Autodesk Fusion 360 part; units mm, degrees
note: some values were not read from the file. Chosen so that the rebuilt part matches the saved one: which pieces of a blend or face edit are solid. Set by a fixed rule: which sketch regions a step uses.
(part 2 of 3)
  spline S367 degree 3 poles (41.2974, -19.9603) (42.5718, -19.3541) (43.9034, -18.9073) (45.3289, -18.8182) knots 0 0 0 0 1 1 1 1
  spline S368 degree 3 poles (45.3289, -18.8182) (46.5961, -18.7389) (47.768, -19.0007) (48.7702, -19.8267) knots 0 0 0 0 1 1 1 1
  spline S369 degree 3 poles (48.7702, -19.8267) (49.4912, -20.4209) (49.8984, -21.1818) (49.9641, -22.1189) knots 0 0 0 0 1 1 1 1
  spline S370 degree 3 poles (49.9641, -22.1189) (49.9692, -22.1925) (49.9778, -22.2661) (49.9884, -22.3391) knots 0 0 0 0 1 1 1 1
  spline S371 degree 3 poles (49.9884, -22.3391) (49.9927, -22.3689) (50.0063, -22.3974) (50.0157, -22.4264) knots 0 0 0 0 1 1 1 1
  spline S372 degree 3 poles (50.0157, -22.4264) (50.0388, -22.4327) (50.0618, -22.439) (50.0849, -22.4264) knots 0 0 0 0 1 1 1 1
  spline S373 degree 3 poles (103.7652, -25.3114) (103.6868, -24.832) (103.6099, -23.932) (103.3842, -23.071) knots 0 0 0 0 1 1 1 1
  spline S374 degree 3 poles (103.3842, -23.071) (102.9323, -21.3472) (101.8898, -20.1667) (100.0685, -19.7927) knots 0 0 0 0 1 1 1 1
  spline S375 degree 3 poles (100.0685, -19.7927) (97.9906, -19.366) (96.1141, -19.7496) (94.434, -21.0869) knots 0 0 0 0 1 1 1 1
  spline S376 degree 3 poles (94.434, -21.0869) (92.8843, -22.3203) (91.7133, -23.8561) (90.75, -25.561) knots 0 0 0 0 1 1 1 1
  spline S377 degree 3 poles (90.75, -25.561) (88.9387, -28.7669) (87.8127, -32.2136) (87.2249, -35.8387) knots 0 0 0 0 1 1 1 1
  spline S378 degree 3 poles (87.2249, -35.8387) (86.9707, -37.4063) (86.8196, -38.9843) (87.089, -40.569) knots 0 0 0 0 1 1 1 1
  spline S379 degree 3 poles (87.089, -40.569) (87.4308, -42.5797) (88.511, -43.9928) (90.5089, -44.5579) knots 0 0 0 0 1 1 1 1
  spline S380 degree 3 poles (90.5089, -44.5579) (92.2381, -45.047) (93.88, -44.7412) (95.3927, -43.7705) knots 0 0 0 0 1 1 1 1
  spline S381 degree 3 poles (95.3927, -43.7705) (96.8708, -42.822) (98.0012, -41.534) (98.9616, -40.0853) knots 0 0 0 0 1 1 1 1
  spline S382 degree 3 poles (98.9616, -40.0853) (100.7237, -37.4275) (101.8987, -34.5089) (102.7607, -31.4561) knots 0 0 0 0 1 1 1 1
  spline S383 degree 3 poles (102.7607, -31.4561) (103.2897, -29.5826) (103.6858, -27.6833) (103.7652, -25.3114) knots 0 0 0 0 1 1 1 1
  spline S384 degree 3 poles (46.0065, -19.6332) (44.9669, -19.627) (44.0162, -19.8508) (43.1126, -20.2652) knots 0 0 0 0 1 1 1 1
  spline S385 degree 3 poles (43.1126, -20.2652) (41.2513, -21.1186) (39.7466, -22.4329) (38.4102, -23.9545) knots 0 0 0 0 1 1 1 1
  spline S386 degree 3 poles (38.4102, -23.9545) (36.618, -25.9951) (35.2451, -28.3068) (34.0956, -30.753) knots 0 0 0 0 1 1 1 1
  spline S387 degree 3 poles (34.0956, -30.753) (32.774, -33.5658) (31.7466, -36.4734) (31.4534, -39.5941) knots 0 0 0 0 1 1 1 1
  spline S388 degree 3 poles (31.4534, -39.5941) (31.3429, -40.7711) (31.3958, -41.9355) (31.8603, -43.0504) knots 0 0 0 0 1 1 1 1
  spline S389 degree 3 poles (31.8603, -43.0504) (32.3368, -44.1941) (33.2068, -44.7345) (34.4271, -44.7672) knots 0 0 0 0 1 1 1 1
  spline S390 degree 3 poles (34.4271, -44.7672) (35.6477, -44.7998) (36.7623, -44.4442) (37.8098, -43.852) knots 0 0 0 0 1 1 1 1
  spline S391 degree 3 poles (37.8098, -43.852) (40.0373, -42.5928) (41.8175, -40.8319) (43.3761, -38.8332) knots 0 0 0 0 1 1 1 1
  spline S392 degree 3 poles (43.3761, -38.8332) (44.1228, -37.8756) (44.8434, -36.8973) (45.2618, -35.7354) knots 0 0 0 0 1 1 1 1
  spline S393 degree 3 poles (45.2618, -35.7354) (46.3267, -32.778) (47.4017, -29.8244) (48.4649, -26.8664) knots 0 0 0 0 1 1 1 1
  spline S394 degree 3 poles (48.4649, -26.8664) (48.8497, -25.7959) (49.3037, -24.7413) (49.4107, -23.5928) knots 0 0 0 0 1 1 1 1
  spline S395 degree 3 poles (49.4107, -23.5928) (49.6232, -21.3105) (48.1691, -19.514) (46.0065, -19.6332) knots 0 0 0 0 1 1 1 1
  spline S396 degree 3 poles (84.1667, -10.1913) (84.1729, -8.6259) (85.3768, -7.4326) (86.9503, -7.4324) knots 0 0 0 0 1 1 1 1
  spline S397 degree 3 poles (86.9503, -7.4324) (88.5314, -7.4321) (89.7239, -8.6369) (89.7211, -10.2316) knots 0 0 0 0 1 1 1 1
  spline S398 degree 3 poles (89.7211, -10.2316) (89.7183, -11.8206) (88.5136, -13.0149) (86.9258, -13.0029) knots 0 0 0 0 1 1 1 1
  spline S399 degree 3 poles (86.9258, -13.0029) (85.3374, -12.9908) (84.1605, -11.7915) (84.1667, -10.1913) knots 0 0 0 0 1 1 1 1
  spline S400 degree 3 poles (128.8614, -26.1716) (128.8153, -28.284) (128.276, -30.6235) (127.5153, -32.9166) knots 0 0 0 0 1 1 1 1
  spline S401 degree 3 poles (127.5153, -32.9166) (126.5931, -35.6965) (125.3817, -38.3368) (123.61, -40.6911) knots 0 0 0 0 1 1 1 1
  spline S402 degree 3 poles (123.61, -40.6911) (122.5647, -42.0801) (121.3489, -43.2903) (119.806, -44.129) knots 0 0 0 0 1 1 1 1
  spline S403 degree 3 poles (119.806, -44.129) (118.0331, -45.0928) (115.4801, -45.0947) (113.845, -43.5861) knots 0 0 0 0 1 1 1 1
  spline S404 degree 3 poles (113.845, -43.5861) (112.9324, -42.7442) (112.3341, -41.7221) (111.9863, -40.5443) knots 0 0 0 0 1 1 1 1
  spline S405 degree 3 poles (111.9863, -40.5443) (111.834, -40.0287) (111.687, -39.5095) (111.5818, -38.983) knots 0 0 0 0 1 1 1 1
  spline S406 degree 3 poles (111.5818, -38.983) (111.5353, -38.7499) (111.5424, -38.4751) (111.6206, -38.2527) knots 0 0 0 0 1 1 1 1
  spline S407 degree 3 poles (111.6206, -38.2527) (113.0797, -34.1034) (114.5515, -29.9585) (116.0281, -25.8153) knots 0 0 0 0 1 1 1 1
  spline S408 degree 3 poles (116.0281, -25.8153) (116.1079, -25.5914) (116.2291, -25.3728) (116.3717, -25.182) knots 0 0 0 0 1 1 1 1
  spline S409 degree 3 poles (116.3717, -25.182) (117.2705, -23.9794) (118.185, -22.7878) (119.3159, -21.7871) knots 0 0 0 0 1 1 1 1
  spline S410 degree 3 poles (119.3159, -21.7871) (120.4047, -20.8235) (121.5941, -20.0336) (123.056, -19.7578) knots 0 0 0 0 1 1 1 1
  spline S411 degree 3 poles (123.056, -19.7578) (123.9276, -19.5934) (124.8028, -19.5937) (125.6676, -19.8061) knots 0 0 0 0 1 1 1 1
  spline S412 degree 3 poles (125.6676, -19.8061) (126.9085, -20.111) (127.6838, -20.9266) (128.1613, -22.0809) knots 0 0 0 0 1 1 1 1
  spline S413 degree 3 poles (128.1613, -22.0809) (128.6621, -23.2915) (128.8638, -24.5521) (128.8614, -26.1716) knots 0 0 0 0 1 1 1 1
  spline S414 degree 3 poles (138.7712, -30.0038) (139.2283, -29.0291) (139.6235, -28.0968) (140.0927, -27.2034) knots 0 0 0 0 1 1 1 1
  spline S415 degree 3 poles (140.0927, -27.2034) (141.2378, -25.0227) (142.6739, -23.0631) (144.619, -21.5155) knots 0 0 0 0 1 1 1 1
  spline S416 degree 3 poles (144.619, -21.5155) (145.6449, -20.6992) (146.7387, -19.9808) (148.0608, -19.7806) knots 0 0 0 0 1 1 1 1
  spline S417 degree 3 poles (148.0608, -19.7806) (148.7512, -19.6761) (149.4761, -19.6581) (150.1687, -19.7408) knots 0 0 0 0 1 1 1 1
  spline S418 degree 3 poles (150.1687, -19.7408) (151.3327, -19.8797) (152.1161, -20.7367) (152.2726, -21.9102) knots 0 0 0 0 1 1 1 1
  spline S419 degree 3 poles (152.2726, -21.9102) (152.4727, -23.4101) (151.9809, -24.7224) (151.122, -25.9174) knots 0 0 0 0 1 1 1 1
  spline S420 degree 3 poles (151.122, -25.9174) (149.935, -27.569) (148.2949, -28.6145) (146.4395, -29.3662) knots 0 0 0 0 1 1 1 1
  spline S421 degree 3 poles (146.4395, -29.3662) (144.4026, -30.1915) (142.2832, -30.356) (140.1191, -30.1628) knots 0 0 0 0 1 1 1 1
  spline S422 degree 3 poles (140.1191, -30.1628) (139.7002, -30.1254) (139.2833, -30.0649) (138.7712, -30.0038) knots 0 0 0 0 1 1 1 1
  spline S423 degree 3 poles (103.7652, -25.3302) (103.6859, -27.7021) (103.2897, -29.6014) (102.7607, -31.4749) knots 0 0 0 0 1 1 1 1
  spline S424 degree 3 poles (102.7607, -31.4749) (101.8987, -34.5277) (100.7238, -37.4463) (98.9617, -40.1041) knots 0 0 0 0 1 1 1 1
  spline S425 degree 3 poles (98.9617, -40.1041) (98.0012, -41.5528) (96.8709, -42.8408) (95.3927, -43.7893) knots 0 0 0 0 1 1 1 1
  spline S426 degree 3 poles (95.3927, -43.7893) (93.8801, -44.76) (92.2382, -45.0658) (90.509, -44.5767) knots 0 0 0 0 1 1 1 1
  spline S427 degree 3 poles (90.509, -44.5767) (88.511, -44.0116) (87.4309, -42.5985) (87.089, -40.5878) knots 0 0 0 0 1 1 1 1
  spline S428 degree 3 poles (87.089, -40.5878) (86.8196, -39.0031) (86.9707, -37.4251) (87.2249, -35.8575) knots 0 0 0 0 1 1 1 1
  spline S429 degree 3 poles (87.2249, -35.8575) (87.8128, -32.2324) (88.9387, -28.7857) (90.7501, -25.5798) knots 0 0 0 0 1 1 1 1
  spline S430 degree 3 poles (90.7501, -25.5798) (91.7133, -23.8749) (92.8844, -22.3391) (94.4341, -21.1057) knots 0 0 0 0 1 1 1 1
  spline S431 degree 3 poles (94.4341, -21.1057) (96.1142, -19.7684) (97.9907, -19.3848) (100.0686, -19.8115) knots 0 0 0 0 1 1 1 1
  spline S432 degree 3 poles (100.0686, -19.8115) (101.8899, -20.1855) (102.9323, -21.366) (103.3842, -23.0898) knots 0 0 0 0 1 1 1 1
  spline S433 degree 3 poles (103.3842, -23.0898) (103.61, -23.9508) (103.6869, -24.8508) (103.7652, -25.3302) knots 0 0 0 0 1 1 1 1
  spline S434 degree 3 poles (46.0066, -19.652) (48.1692, -19.5328) (49.6232, -21.3293) (49.4107, -23.6116) knots 0 0 0 0 1 1 1 1
  spline S435 degree 3 poles (49.4107, -23.6116) (49.3038, -24.7601) (48.8497, -25.8147) (48.4649, -26.8852) knots 0 0 0 0 1 1 1 1
  spline S436 degree 3 poles (48.4649, -26.8852) (47.4017, -29.8432) (46.3267, -32.7968) (45.2618, -35.7542) knots 0 0 0 0 1 1 1 1
  spline S437 degree 3 poles (45.2618, -35.7542) (44.8434, -36.9161) (44.1228, -37.8944) (43.3761, -38.852) knots 0 0 0 0 1 1 1 1
  spline S438 degree 3 poles (43.3761, -38.852) (41.8175, -40.8507) (40.0373, -42.6116) (37.8099, -43.8708) knots 0 0 0 0 1 1 1 1
  spline S439 degree 3 poles (37.8099, -43.8708) (36.7624, -44.463) (35.6477, -44.8186) (34.4271, -44.786) knots 0 0 0 0 1 1 1 1
  spline S440 degree 3 poles (34.4271, -44.786) (33.2068, -44.7533) (32.3368, -44.213) (31.8603, -43.0692) knots 0 0 0 0 1 1 1 1
  spline S441 degree 3 poles (31.8603, -43.0692) (31.3958, -41.9543) (31.3429, -40.7899) (31.4535, -39.6129) knots 0 0 0 0 1 1 1 1
  spline S442 degree 3 poles (31.4535, -39.6129) (31.7466, -36.4922) (32.774, -33.5846) (34.0957, -30.7718) knots 0 0 0 0 1 1 1 1
  spline S443 degree 3 poles (34.0957, -30.7718) (35.2451, -28.3256) (36.618, -26.0139) (38.4102, -23.9733) knots 0 0 0 0 1 1 1 1
  spline S444 degree 3 poles (38.4102, -23.9733) (39.7466, -22.4517) (41.2513, -21.1374) (43.1126, -20.284) knots 0 0 0 0 1 1 1 1
  spline S445 degree 3 poles (43.1126, -20.284) (44.0162, -19.8697) (44.967, -19.6458) (46.0066, -19.652) knots 0 0 0 0 1 1 1 1
extrude "Extrude3" add sketch "Sketch3" along normal blind 6.35 contours S23 S24 S25 S26 S27 S28 S29 S30 S31 S32 S33 S34 S35 S36 S37 S38 S39 S40 S41 S42 S43 S44 S45 S214 S215 S216 S217 S218 S219 S220 S221 S222 S223 S224 S225 S226 S227 S228 S229 S230 S231 S232 S233 S234 S235 L21 | S0 L2 S1 S2 S3 S4 S5 S6 S7 S8 S9 S10 L3 S11 L4 S12 S13 S14 S15 L5 S16 S17 S18 S19 S20 S21 S178 S179 S180 S181 S182 S183 L16 S184 S185 S186 S187 L17 S188 L18 S189 S190 S191 S192 S193 S194 S195 S196 S197 S198 L19 S199 L20 | S46 S47 S48 S49 S50 S51 S52 S53 S54 S55 S56 S57 S58 S59 S60 S61 S62 S63 S64 S65 S66 S67 S68 S69 S70 S71 S72 S73 S74 S75 S76 S77 S78 S79 S80 S81 S82 S83 S84 S85 S86 S87 S88 S89 S90 S91 S92 S93 S94 S95 S96 S97 S98 S99 S100 S101 S102 S103 S104 S105 S106 S107 S108 S109 S111 S112 S113 S114 S115 S116 S117 S118 S119 S120 S121 S122 S123 S124 S125 S126 S127 S128 L9 S129 S130 S131 S132 L10 S133 S134 S135 S136 S137 S138 S139 S140 S141 S142 L11 S143 S144 S145 L12 S146 S147 S148 S149 S150 S151 S152 S153 S154 S155 L13 S156 L14 S157 S158 S159 S160 S161 S162 S163 S164 S165 S166 S167 S168 S169 S170 S171 S172 S173 S245 S246 S247 S248 S249 S250 S251 S252 S253 S254 S255 S256 S257 S258 S259 S260 S261 L22 S262 L23 S263 S264 S265 S266 S267 S268 S269 S270 S271 S272 L24 S273 S274 S275 L25 S276 S277 S278 S279 S280 S281 S282 S283 S284 S285 L26 S286 S287 S288 S289 L27 S290 S291 S292 S293 S294 S295 S296 S297 S298 S299 S300 S301 S302 S303 S304 S305 S306 S307 S309 S310 S311 S312 S313 S314 S315 S316 S317 S318 S319 S320 S321 S322 S323 S324 S325 S326 S327 S328 S329 S330 S331 S332 S333 S334 S335 S336 S337 S338 S339 S340 S341 S342 S343 S344 S345 S346 S347 S348 S349 S350 S351 S352 S353 S354 S355 S356 S357 S358 S359 S360 S361 S362 S363 S364 S365 S366 S367 S368 S369 S370 S371 | S174 S175 S176 S177 S396 S397 S398 S399 makes body 1 at (108.0941, -40.2976, 0) makes body 2 at (65.2632, -12.3093, 0) makes body 3 at (138.449, -28.0132, 0) makes body 4 at (84.2074, -10.7088, 2.8222)
sketch "Sketch4" plane through (0, 0, 0) normal (0, 0, 1) x (1, 0, 0)
  line L0 (0, 0) -> (156.0835, 0)
  line L1 (156.0835, 0) -> (156.0835, -61.3211)
  line L2 (156.0835, -61.3211) -> (0, -61.3211)
  line L3 (0, -61.3211) -> (0, 0)
  constraint horizontal L0
  constraint vertical L1
  constraint horizontal L2
  constraint vertical L3
  constraint coincident L0.start L3.end
extrude "Extrude4" add sketch "Sketch4" against normal blind 6.35 bodies 1 2 3 4
fillet "Fillet1" radius 6.35 4 edges at (0, -61.3211, -3.175) (156.0835, -61.3211, -3.175) (156.0835, 0, -3.175) (0, 0, -3.175) on bodies 1
sketch "Sketch1" plane through (0, 0, 0) normal (0, 0, 1) x (1, 0, 0)
  line L0 (156.0195, -23.5976) -> (156.0195, -61.341)
  line L1 (156.0195, -61.341) -> (108.4773, -61.341)
  spline S0 degree 3 poles (108.4773, -61.341) (108.5491, -61.0596) (108.6209, -60.7783) (108.7043, -60.4516) knots 0 0 0 0 1 1 1 1
  line L2 (108.7043, -60.4516) -> (103.7692, -60.4516)
  spline S1 degree 3 poles (103.7692, -60.4516) (106.1753, -53.6131) (108.5658, -46.8189) (110.9796, -39.9584) knots 0 0 0 0 1 1 1 1
  spline S2 degree 3 poles (110.9796, -39.9584) (111.1778, -40.6135) (111.3001, -41.1945) (111.5257, -41.7321) knots 0 0 0 0 1 1 1 1
  spline S3 degree 3 poles (111.5257, -41.7321) (112.4488, -43.9326) (114.0522, -45.3171) (116.4762, -45.532) knots 0 0 0 0 1 1 1 1
  spline S4 degree 3 poles (116.4762, -45.532) (118.5105, -45.7123) (120.4877, -45.3426) (122.343, -44.485) knots 0 0 0 0 1 1 1 1
  spline S5 degree 3 poles (122.343, -44.485) (125.9058, -42.8382) (128.6456, -40.264) (130.6312, -36.8985) knots 0 0 0 0 1 1 1 1
  spline S6 degree 3 poles (130.6312, -36.8985) (132.3382, -34.0054) (133.3231, -30.9198) (132.9158, -27.5036) knots 0 0 0 0 1 1 1 1
  spline S7 degree 3 poles (132.9158, -27.5036) (132.7164, -25.831) (132.2982, -24.2283) (131.4403, -22.7614) knots 0 0 0 0 1 1 1 1
  spline S8 degree 3 poles (131.4403, -22.7614) (129.2488, -19.0142) (125.0975, -18.1221) (121.9017, -19.2309) knots 0 0 0 0 1 1 1 1
  spline S9 degree 3 poles (121.9017, -19.2309) (119.7817, -19.9664) (118.1223, -21.3511) (116.8137, -23.1628) knots 0 0 0 0 1 1 1 1
  spline S10 degree 3 poles (116.8137, -23.1628) (116.7552, -23.2438) (116.6934, -23.3224) (116.6331, -23.4021) knots 0 0 0 0 1 1 1 1
  line L3 (116.6331, -23.4021) -> (116.5718, -23.3725)
  spline S11 degree 3 poles (116.5718, -23.3725) (116.9751, -22.1176) (117.3783, -20.8626) (117.794, -19.5691) knots 0 0 0 0 1 1 1 1
  line L4 (117.794, -19.5691) -> (117.39, -19.5691)
  spline S12 degree 3 poles (117.39, -19.5691) (116.1524, -19.5691) (114.9147, -19.5691) (113.677, -19.5691) knots 0 0 0 0 1 1 1 1
  spline S13 degree 3 poles (113.677, -19.5691) (112.0374, -19.5691) (110.3977, -19.567) (108.7581, -19.5739) knots 0 0 0 0 1 1 1 1
  spline S14 degree 3 poles (108.7581, -19.5739) (108.6477, -19.5743) (108.4711, -19.6131) (108.4397, -19.6844) knots 0 0 0 0 1 1 1 1
  spline S15 degree 3 poles (108.4397, -19.6844) (108.3413, -19.9076) (108.2979, -20.1549) (108.2252, -20.4221) knots 0 0 0 0 1 1 1 1
  line L5 (108.2252, -20.4221) -> (113.6878, -20.4221)
  spline S16 degree 3 poles (113.6878, -20.4221) (113.6473, -20.5473) (113.6177, -20.6465) (113.5834, -20.7441) knots 0 0 0 0 1 1 1 1
  spline S17 degree 3 poles (113.5834, -20.7441) (108.9605, -33.8922) (104.3365, -47.04) (99.7194, -60.1902) knots 0 0 0 0 1 1 1 1
  spline S18 degree 3 poles (99.7194, -60.1902) (99.6414, -60.4125) (99.533, -60.4699) (99.3115, -60.4681) knots 0 0 0 0 1 1 1 1
  spline S19 degree 3 poles (99.3115, -60.4681) (98.0845, -60.4581) (96.8573, -60.46) (95.6303, -60.4696) knots 0 0 0 0 1 1 1 1
  spline S20 degree 3 poles (95.6303, -60.4696) (95.5302, -60.4704) (95.3717, -60.5363) (95.342, -60.6118) knots 0 0 0 0 1 1 1 1
  spline S21 degree 3 poles (95.342, -60.6118) (95.2508, -60.8445) (95.2089, -61.0965) (95.1478, -61.341) knots 0 0 0 0 1 1 1 1
  line L6 (95.1478, -61.341) -> (0, -61.341)
  line L7 (0, -61.341) -> (0, 0)
  spline S22 degree 3 poles (0, 0) (52.0065, 0) (104.013, 0) (156.0195, 0) knots 0 0 0 0 1 1 1 1
  line L8 (156.0195, 0) -> (156.0195, -22.8998)
  spline S23 degree 3 poles (156.0195, -22.8998) (156.0019, -22.8646) (155.9715, -22.8305) (155.9685, -22.7942) knots 0 0 0 0 1 1 1 1
  spline S24 degree 3 poles (155.9685, -22.7942) (155.8892, -21.8192) (155.4189, -21.052) (154.6851, -20.4397) knots 0 0 0 0 1 1 1 1
  spline S25 degree 3 poles (154.6851, -20.4397) (153.4053, -19.3719) (151.8701, -18.9809) (150.2562, -18.8437) knots 0 0 0 0 1 1 1 1
  spline S26 degree 3 poles (150.2562, -18.8437) (147.8053, -18.6354) (145.5366, -19.2454) (143.4312, -20.4739) knots 0 0 0 0 1 1 1 1
  spline S27 degree 3 poles (143.4312, -20.4739) (139.1005, -23.0008) (136.0205, -26.6341) (134.0532, -31.2182) knots 0 0 0 0 1 1 1 1
  spline S28 degree 3 poles (134.0532, -31.2182) (133.1018, -33.4352) (132.6126, -35.7441) (132.9818, -38.1701) knots 0 0 0 0 1 1 1 1
  spline S29 degree 3 poles (135.3221, -43.0231) (136.8021, -44.5156) (138.6131, -45.3113) (140.7013, -45.5057) knots 0 0 0 0 1 1 1 1
  spline S30 degree 3 poles (140.7013, -45.5057) (143.1519, -45.7339) (145.4639, -45.3818) (147.6206, -44.0951) knots 0 0 0 0 1 1 1 1
  spline S31 degree 3 poles (147.6206, -44.0951) (149.696, -42.8569) (151.1962, -41.1095) (152.41, -39.0493) knots 0 0 0 0 1 1 1 1
  spline S32 degree 3 poles (152.41, -39.0493) (152.1937, -38.9254) (151.9691, -38.7968) (151.7296, -38.6596) knots 0 0 0 0 1 1 1 1
  spline S33 degree 3 poles (151.7296, -38.6596) (151.52, -38.9343) (151.3182, -39.1785) (151.1384, -39.4379) knots 0 0 0 0 1 1 1 1
  spline S34 degree 3 poles (151.1384, -39.4379) (150.286, -40.6676) (149.3449, -41.8167) (148.1741, -42.7628) knots 0 0 0 0 1 1 1 1
  spline S35 degree 3 poles (148.1741, -42.7628) (146.3193, -44.2615) (144.246, -45.0682) (141.8277, -44.718) knots 0 0 0 0 1 1 1 1
  spline S36 degree 3 poles (141.8277, -44.718) (139.955, -44.4468) (138.4938, -43.5447) (137.642, -41.8068) knots 0 0 0 0 1 1 1 1
  spline S37 degree 3 poles (137.642, -41.8068) (137.1687, -40.8411) (137.0345, -39.7935) (137.0087, -38.7285) knots 0 0 0 0 1 1 1 1
  spline S38 degree 3 poles (137.0087, -38.7285) (136.9596, -36.7106) (137.328, -34.757) (137.9094, -32.836) knots 0 0 0 0 1 1 1 1
  spline S39 degree 3 poles (137.9094, -32.836) (138.1099, -32.1735) (138.3185, -31.5134) (138.503, -30.9178) knots 0 0 0 0 1 1 1 1
  spline S40 degree 3 poles (138.503, -30.9178) (139.7894, -30.9729) (141.0146, -31.0989) (142.2347, -31.0619) knots 0 0 0 0 1 1 1 1
  spline S41 degree 3 poles (142.2347, -31.0619) (144.493, -30.9934) (146.7045, -30.5779) (148.8648, -29.9105) knots 0 0 0 0 1 1 1 1
  spline S42 degree 3 poles (148.8648, -29.9105) (150.5076, -29.403) (152.0871, -28.7496) (153.4759, -27.7167) knots 0 0 0 0 1 1 1 1
  spline S43 degree 3 poles (153.4759, -27.7167) (154.6089, -26.874) (155.5238, -25.8533) (155.8582, -24.4251) knots 0 0 0 0 1 1 1 1
  spline S44 degree 3 poles (155.8582, -24.4251) (155.9223, -24.1517) (155.9663, -23.8735) (156.0195, -23.5976) knots 0 0 0 0 1 1 1 1
  spline S45 degree 3 poles (50.0849, -22.4452) (50.0619, -22.439) (50.0388, -22.4327) (50.0158, -22.4265) knots 0 0 0 0 1 1 1 1
  spline S46 degree 3 poles (50.0158, -22.4265) (50.0064, -22.3974) (49.9927, -22.3689) (49.9884, -22.3392) knots 0 0 0 0 1 1 1 1
  spline S47 degree 3 poles (49.9884, -22.3392) (49.9779, -22.2661) (49.9693, -22.1925) (49.9641, -22.1189) knots 0 0 0 0 1 1 1 1
  spline S48 degree 3 poles (49.9641, -22.1189) (49.8984, -21.1818) (49.4912, -20.4209) (48.7702, -19.8267) knots 0 0 0 0 1 1 1 1
  spline S49 degree 3 poles (48.7702, -19.8267) (47.7681, -19.0007) (46.5961, -18.7389) (45.3289, -18.8182) knots 0 0 0 0 1 1 1 1
  spline S50 degree 3 poles (45.3289, -18.8182) (43.9034, -18.9073) (42.5718, -19.3541) (41.2975, -19.9603) knots 0 0 0 0 1 1 1 1
  spline S51 degree 3 poles (41.2975, -19.9603) (37.4617, -21.785) (34.2471, -24.4068) (31.5841, -27.6967) knots 0 0 0 0 1 1 1 1
  spline S52 degree 3 poles (31.5841, -27.6967) (29.8681, -29.8167) (28.5608, -32.172) (27.7761, -34.8009) knots 0 0 0 0 1 1 1 1
  spline S53 degree 3 poles (27.7761, -34.8009) (27.6548, -35.2071) (27.6013, -35.6146) (27.2979, -35.9909) knots 0 0 0 0 1 1 1 1
  spline S54 degree 3 poles (27.2979, -35.9909) (26.7981, -36.6105) (26.4452, -37.3469) (26.0145, -38.024) knots 0 0 0 0 1 1 1 1
  spline S55 degree 3 poles (26.0145, -38.024) (24.3785, -40.5957) (22.1935, -42.5594) (19.4153, -43.8207) knots 0 0 0 0 1 1 1 1
  spline S56 degree 3 poles (19.4153, -43.8207) (16.336, -45.2186) (13.1649, -45.1705) (10.0109, -44.1478) knots 0 0 0 0 1 1 1 1
  spline S57 degree 3 poles (10.0109, -44.1478) (7.3021, -43.2695) (5.6053, -41.3794) (4.9304, -38.5933) knots 0 0 0 0 1 1 1 1
  spline S58 degree 3 poles (4.9304, -38.5933) (4.4781, -36.726) (4.5193, -34.842) (4.7229, -32.9543) knots 0 0 0 0 1 1 1 1
  spline S59 degree 3 poles (4.7229, -32.9543) (5.0136, -30.2599) (5.5761, -27.6183) (6.3535, -25.0241) knots 0 0 0 0 1 1 1 1
  spline S60 degree 3 poles (6.3535, -25.0241) (7.7161, -20.4766) (9.4965, -16.1067) (12.0128, -12.064) knots 0 0 0 0 1 1 1 1
  spline S61 degree 3 poles (12.0128, -12.064) (13.6498, -9.4342) (15.5983, -7.0752) (18.1065, -5.2075) knots 0 0 0 0 1 1 1 1
  spline S62 degree 3 poles (18.1065, -5.2075) (21.6115, -2.5974) (25.4024, -2.3618) (29.3636, -3.8873) knots 0 0 0 0 1 1 1 1
  spline S63 degree 3 poles (29.3636, -3.8873) (31.4072, -4.6744) (32.7504, -6.1919) (33.298, -8.3429) knots 0 0 0 0 1 1 1 1
  spline S64 degree 3 poles (33.298, -8.3429) (33.6344, -9.6642) (33.5355, -11.0084) (33.4161, -12.3468) knots 0 0 0 0 1 1 1 1
  spline S65 degree 3 poles (33.4161, -12.3468) (33.3593, -12.9843) (33.2661, -13.6185) (33.1895, -14.2539) knots 0 0 0 0 1 1 1 1
  spline S66 degree 3 poles (33.1895, -14.2539) (33.924, -14.3486) (33.9218, -14.3478) (34.1497, -13.71) knots 0 0 0 0 1 1 1 1
  spline S67 degree 3 poles (34.1497, -13.71) (35.1509, -10.908) (36.1535, -8.1065) (37.1555, -5.3048) knots 0 0 0 0 1 1 1 1
  spline S68 degree 3 poles (37.1555, -5.3048) (37.4387, -4.513) (37.7215, -3.721) (38.014, -2.9026) knots 0 0 0 0 1 1 1 1
  spline S69 degree 3 poles (38.014, -2.9026) (37.8301, -2.8616) (37.6735, -2.8421) (37.5281, -2.7909) knots 0 0 0 0 1 1 1 1
  spline S70 degree 3 poles (37.5281, -2.7909) (37.2322, -2.6868) (37.0752, -2.7732) (36.9084, -3.0554) knots 0 0 0 0 1 1 1 1
  spline S71 degree 3 poles (36.9084, -3.0554) (36.3629, -3.9783) (35.5622, -4.5251) (34.4509, -4.4166) knots 0 0 0 0 1 1 1 1
  spline S72 degree 3 poles (34.4509, -4.4166) (33.9099, -4.3637) (33.3658, -4.2376) (32.8488, -4.0667) knots 0 0 0 0 1 1 1 1
  spline S73 degree 3 poles (32.8488, -4.0667) (31.9676, -3.7753) (31.1102, -3.4127) (30.2365, -3.0973) knots 0 0 0 0 1 1 1 1
  spline S74 degree 3 poles (30.2365, -3.0973) (27.7778, -2.2096) (25.2539, -1.9088) (22.6573, -2.2749) knots 0 0 0 0 1 1 1 1
  spline S75 degree 3 poles (22.6573, -2.2749) (20.7362, -2.5458) (18.9175, -3.1537) (17.1711, -3.9759) knots 0 0 0 0 1 1 1 1
  spline S76 degree 3 poles (17.1711, -3.9759) (11.8716, -6.4708) (7.6391, -10.2081) (4.4487, -15.0988) knots 0 0 0 0 1 1 1 1
  spline S77 degree 3 poles (4.4487, -15.0988) (1.4603, -19.6798) (-0.1988, -24.667) (0.1153, -30.2088) knots 0 0 0 0 1 1 1 1
  spline S78 degree 3 poles (0.1153, -30.2088) (0.2462, -32.5189) (0.589, -34.789) (1.4018, -36.9651) knots 0 0 0 0 1 1 1 1
  spline S79 degree 3 poles (1.4018, -36.9651) (2.7269, -40.5128) (5.07, -43.1219) (8.5869, -44.6156) knots 0 0 0 0 1 1 1 1
  spline S80 degree 3 poles (8.5869, -44.6156) (9.982, -45.2081) (11.4556, -45.483) (12.9615, -45.5794) knots 0 0 0 0 1 1 1 1
  spline S81 degree 3 poles (12.9615, -45.5794) (14.9147, -45.7043) (16.8656, -45.6654) (18.7272, -44.9928) knots 0 0 0 0 1 1 1 1
  spline S82 degree 3 poles (18.7272, -44.9928) (22.1612, -43.7524) (24.8613, -41.5667) (26.8476, -38.5034) knots 0 0 0 0 1 1 1 1
  spline S83 degree 3 poles (26.8476, -38.5034) (26.988, -38.287) (27.118, -38.0638) (27.2529, -37.8437) knots 0 0 0 0 1 1 1 1
  spline S84 degree 3 poles (27.2529, -37.8437) (27.3252, -37.9926) (27.3127, -38.1253) (27.3273, -38.2549) knots 0 0 0 0 1 1 1 1
  spline S85 degree 3 poles (27.3273, -38.2549) (27.4213, -39.0926) (27.4431, -39.948) (27.6348, -40.7633) knots 0 0 0 0 1 1 1 1
  spline S86 degree 3 poles (27.6348, -40.7633) (28.0824, -42.6659) (29.1177, -44.1579) (30.9434, -45.0023) knots 0 0 0 0 1 1 1 1
  spline S87 degree 3 poles (30.9434, -45.0023) (32.3176, -45.6378) (33.7642, -45.6821) (35.2298, -45.4504) knots 0 0 0 0 1 1 1 1
  spline S88 degree 3 poles (35.2298, -45.4504) (37.0632, -45.1607) (38.6343, -44.293) (40.0946, -43.1941) knots 0 0 0 0 1 1 1 1
  spline S89 degree 3 poles (40.0946, -43.1941) (41.6556, -42.0196) (42.8844, -40.5225) (44.1283, -39.0402) knots 0 0 0 0 1 1 1 1
  spline S90 degree 3 poles (44.1283, -39.0402) (44.2114, -38.9412) (44.2975, -38.8447) (44.3823, -38.747) knots 0 0 0 0 1 1 1 1
  spline S91 degree 3 poles (44.3823, -38.747) (44.4123, -38.9053) (44.3802, -39.0239) (44.3478, -39.1425) knots 0 0 0 0 1 1 1 1
  spline S92 degree 3 poles (44.3478, -39.1425) (44.0412, -40.2656) (43.7805, -41.3953) (43.8608, -42.5731) knots 0 0 0 0 1 1 1 1
  spline S93 degree 3 poles (43.8608, -42.5731) (43.9596, -44.0239) (44.7538, -45.0434) (46.147, -45.3786) knots 0 0 0 0 1 1 1 1
  spline S94 degree 3 poles (46.147, -45.3786) (47.775, -45.7703) (49.3655, -45.6409) (50.8342, -44.773) knots 0 0 0 0 1 1 1 1
  spline S95 degree 3 poles (50.8342, -44.773) (51.4483, -44.4101) (52.0194, -43.9749) (52.6073, -43.5745) knots 0 0 0 0 1 1 1 1
  spline S96 degree 3 poles (52.6073, -43.5745) (53.0764, -44.5495) (53.5786, -45.0228) (54.6679, -45.2941) knots 0 0 0 0 1 1 1 1
  spline S97 degree 3 poles (54.6679, -45.2941) (55.3375, -45.4608) (56.041, -45.5543) (56.731, -45.5649) knots 0 0 0 0 1 1 1 1
  spline S98 degree 3 poles (56.731, -45.5649) (58.821, -45.5971) (60.4965, -44.6726) (61.8903, -43.1798) knots 0 0 0 0 1 1 1 1
  spline S99 degree 3 poles (61.8903, -43.1798) (62.2327, -42.813) (62.5336, -42.4076) (62.8925, -41.9728) knots 0 0 0 0 1 1 1 1
  spline S100 degree 3 poles (62.8925, -41.9728) (62.8925, -42.1445) (62.8903, -42.2662) (62.8928, -42.3877) knots 0 0 0 0 1 1 1 1
  spline S101 degree 3 poles (62.8928, -42.3877) (62.9231, -43.8262) (63.5858, -44.7511) (64.9382, -45.2356) knots 0 0 0 0 1 1 1 1
  spline S102 degree 3 poles (64.9382, -45.2356) (65.967, -45.6042) (67.0307, -45.6375) (68.0997, -45.5148) knots 0 0 0 0 1 1 1 1
  spline S103 degree 3 poles (68.0997, -45.5148) (69.8832, -45.31) (71.2784, -44.3806) (72.4656, -43.096) knots 0 0 0 0 1 1 1 1
  spline S104 degree 3 poles (72.4656, -43.096) (72.7758, -42.7603) (73.0458, -42.3875) (73.3767, -41.9795) knots 0 0 0 0 1 1 1 1
  spline S105 degree 3 poles (73.3767, -41.9795) (73.3767, -42.1348) (73.3743, -42.2262) (73.3771, -42.3173) knots 0 0 0 0 1 1 1 1
  spline S106 degree 3 poles (73.3771, -42.3173) (73.4271, -43.9443) (74.2035, -44.9618) (75.7898, -45.3455) knots 0 0 0 0 1 1 1 1
  spline S107 degree 3 poles (75.7898, -45.3455) (78.4926, -45.9992) (80.8441, -45.3252) (82.7546, -43.3024) knots 0 0 0 0 1 1 1 1
  spline S108 degree 3 poles (82.7546, -43.3024) (83.3917, -42.6279) (83.8997, -41.8316) (84.4745, -41.0809) knots 0 0 0 0 1 1 1 1
  spline S109 degree 3 poles (84.4745, -41.0809) (84.4258, -41.054) (84.4504, -41.0594) (84.4605, -41.0746) knots 0 0 0 0 1 1 1 1
  spline S110 degree 3 poles (84.4605, -41.0746) (84.5133, -41.1535) (84.5617, -41.2351) (84.6127, -41.3152) knots 0 0 0 0 1 1 1 1
  spline S111 degree 3 poles (84.6127, -41.3152) (85.7145, -43.047) (87.2073, -44.3196) (89.1334, -45.0354) knots 0 0 0 0 1 1 1 1
  spline S112 degree 3 poles (89.1334, -45.0354) (91.3614, -45.8636) (93.5987, -45.7048) (95.8081, -44.9373) knots 0 0 0 0 1 1 1 1
  spline S113 degree 3 poles (95.8081, -44.9373) (98.3827, -44.0429) (100.6013, -42.5754) (102.4686, -40.6044) knots 0 0 0 0 1 1 1 1
  spline S114 degree 3 poles (102.4686, -40.6044) (105.1593, -37.7643) (107.0753, -34.5158) (107.5538, -30.5511) knots 0 0 0 0 1 1 1 1
  spline S115 degree 3 poles (107.5538, -30.5511) (107.8486, -28.1077) (107.5188, -25.7593) (106.3628, -23.5722) knots 0 0 0 0 1 1 1 1
  spline S116 degree 3 poles (106.3628, -23.5722) (105.1687, -21.313) (103.3851, -19.714) (100.8692, -19.0689) knots 0 0 0 0 1 1 1 1
  spline S117 degree 3 poles (100.8692, -19.0689) (98.8651, -18.5551) (96.8679, -18.7479) (94.9427, -19.4482) knots 0 0 0 0 1 1 1 1
  spline S118 degree 3 poles (94.9427, -19.4482) (89.5691, -21.4031) (85.9017, -25.1273) (83.9323, -30.4535) knots 0 0 0 0 1 1 1 1
  spline S119 degree 3 poles (83.9323, -30.4535) (82.7766, -33.5787) (82.6174, -36.7855) (83.9032, -39.9585) knots 0 0 0 0 1 1 1 1
  spline S120 degree 3 poles (83.9032, -39.9585) (83.9365, -40.0409) (83.9344, -40.169) (83.893, -40.2456) knots 0 0 0 0 1 1 1 1
  spline S121 degree 3 poles (83.893, -40.2456) (83.0471, -41.8113) (81.9568, -43.1756) (80.4699, -44.1743) knots 0 0 0 0 1 1 1 1
  spline S122 degree 3 poles (80.4699, -44.1743) (80.0606, -44.4492) (79.5647, -44.644) (79.081, -44.7494) knots 0 0 0 0 1 1 1 1
  spline S123 degree 3 poles (79.081, -44.7494) (78.0389, -44.9766) (77.2211, -44.4149) (77.0795, -43.4251) knots 0 0 0 0 1 1 1 1
  spline S124 degree 3 poles (77.0795, -43.4251) (77.0352, -43.1161) (77.0232, -42.7789) (77.0991, -42.4806) knots 0 0 0 0 1 1 1 1
  spline S125 degree 3 poles (77.0991, -42.4806) (77.3431, -41.5214) (77.5918, -40.5594) (77.9153, -39.625) knots 0 0 0 0 1 1 1 1
  spline S126 degree 3 poles (77.9153, -39.625) (80.0449, -33.4733) (82.1947, -27.3287) (84.3372, -21.1815) knots 0 0 0 0 1 1 1 1
  spline S127 degree 3 poles (84.3372, -21.1815) (84.5194, -20.6587) (84.6969, -20.1342) (84.8909, -19.5691) knots 0 0 0 0 1 1 1 1
  line L9 (84.8909, -19.5691) -> (84.4958, -19.5691)
  spline S128 degree 3 poles (84.4958, -19.5691) (83.6071, -19.5691) (82.7185, -19.5691) (81.8299, -19.5691) knots 0 0 0 0 1 1 1 1
  spline S129 degree 3 poles (81.8299, -19.5691) (79.82, -19.5691) (77.81, -19.5675) (75.8, -19.5737) knots 0 0 0 0 1 1 1 1
  spline S130 degree 3 poles (75.8, -19.5737) (75.6902, -19.574) (75.5152, -19.6102) (75.4831, -19.6808) knots 0 0 0 0 1 1 1 1
  spline S131 degree 3 poles (75.4831, -19.6808) (75.3826, -19.9022) (75.336, -20.148) (75.2552, -20.4306) knots 0 0 0 0 1 1 1 1
  line L10 (75.2552, -20.4306) -> (80.4962, -20.4306)
  spline S132 degree 3 poles (80.4962, -20.4306) (80.4479, -20.5681) (80.4134, -20.6665) (80.3788, -20.7648) knots 0 0 0 0 1 1 1 1
  spline S133 degree 3 poles (80.3788, -20.7648) (78.5197, -26.0499) (76.6624, -31.3356) (74.7999, -36.6195) knots 0 0 0 0 1 1 1 1
  spline S134 degree 3 poles (74.7999, -36.6195) (74.4293, -37.6709) (74.1085, -38.7475) (73.6419, -39.7556) knots 0 0 0 0 1 1 1 1
  spline S135 degree 3 poles (73.6419, -39.7556) (72.8455, -41.4761) (71.6905, -42.9385) (70.1463, -44.0705) knots 0 0 0 0 1 1 1 1
  spline S136 degree 3 poles (70.1463, -44.0705) (69.6796, -44.4126) (69.1749, -44.6659) (68.5994, -44.764) knots 0 0 0 0 1 1 1 1
  spline S137 degree 3 poles (68.5994, -44.764) (67.3793, -44.9721) (66.5417, -44.2641) (66.5563, -43.0267) knots 0 0 0 0 1 1 1 1
  spline S138 degree 3 poles (66.5563, -43.0267) (66.5593, -42.7745) (66.5643, -42.5124) (66.6319, -42.2727) knots 0 0 0 0 1 1 1 1
  spline S139 degree 3 poles (66.6319, -42.2727) (66.8922, -41.3499) (67.1403, -40.4209) (67.4606, -39.5181) knots 0 0 0 0 1 1 1 1
  spline S140 degree 3 poles (67.4606, -39.5181) (71.9791, -26.78) (76.5089, -14.0458) (81.0355, -1.3105) knots 0 0 0 0 1 1 1 1
  spline S141 degree 3 poles (81.0355, -1.3105) (81.1791, -0.9064) (81.3172, -0.5003) (81.469, -0.0634) knots 0 0 0 0 1 1 1 1
  line L11 (81.469, -0.0634) -> (81.0443, -0.0634)
  spline S142 degree 3 poles (81.0443, -0.0634) (78.2938, -0.0634) (75.5433, -0.0634) (72.7928, -0.0634) knots 0 0 0 0 1 1 1 1
  spline S143 degree 2 poles (72.7928, -0.0634) (72.0388, -0.0634) (71.87, -0.8059) knots 0 0 0 1 1 1
  spline S144 degree 3 poles (71.87, -0.8059) (71.8656, -0.8253) (71.8729, -0.8474) (71.8772, -0.8969) knots 0 0 0 0 1 1 1 1
  line L12 (71.8772, -0.8969) -> (77.0797, -0.8969)
  spline S145 degree 3 poles (77.0797, -0.8969) (77.0261, -1.0528) (76.9874, -1.1697) (76.946, -1.2857) knots 0 0 0 0 1 1 1 1
  spline S146 degree 3 poles (76.946, -1.2857) (72.7448, -13.0394) (68.5443, -24.7933) (64.3408, -36.5461) knots 0 0 0 0 1 1 1 1
  spline S147 degree 3 poles (64.3408, -36.5461) (63.951, -37.6361) (63.6149, -38.7533) (63.1258, -39.7979) knots 0 0 0 0 1 1 1 1
  spline S148 degree 3 poles (63.1258, -39.7979) (62.2985, -41.5649) (61.1119, -43.0774) (59.4732, -44.176) knots 0 0 0 0 1 1 1 1
  spline S149 degree 3 poles (59.4732, -44.176) (59.0639, -44.4504) (58.5683, -44.6503) (58.0846, -44.749) knots 0 0 0 0 1 1 1 1
  spline S150 degree 3 poles (58.0846, -44.749) (56.8852, -44.9938) (56.0307, -44.2662) (56.0713, -43.0432) knots 0 0 0 0 1 1 1 1
  spline S151 degree 3 poles (56.0713, -43.0432) (56.0896, -42.4913) (56.1806, -41.9219) (56.3538, -41.3986) knots 0 0 0 0 1 1 1 1
  spline S152 degree 3 poles (56.3538, -41.3986) (57.0233, -39.3758) (57.7269, -37.364) (58.4397, -35.3559) knots 0 0 0 0 1 1 1 1
  spline S153 degree 3 poles (58.4397, -35.3559) (62.5801, -23.6925) (66.7268, -12.0314) (70.8707, -0.3694) knots 0 0 0 0 1 1 1 1
  spline S154 degree 3 poles (70.8707, -0.3694) (70.9037, -0.2765) (70.9286, -0.1807) (70.961, -0.0737) knots 0 0 0 0 1 1 1 1
  line L13 (70.961, -0.0737) -> (61.5817, -0.0737)
  spline S155 degree 3 poles (61.5817, -0.0737) (61.5071, -0.3392) (61.434, -0.5992) (61.3495, -0.8998) knots 0 0 0 0 1 1 1 1
  line L14 (61.3495, -0.8998) -> (66.5754, -0.8998)
  spline S156 degree 3 poles (66.5754, -0.8998) (66.5356, -1.0258) (66.5105, -1.1153) (66.4793, -1.2026) knots 0 0 0 0 1 1 1 1
  spline S157 degree 3 poles (66.4793, -1.2026) (63.3253, -10.0253) (60.1699, -18.8474) (57.0169, -27.6704) knots 0 0 0 0 1 1 1 1
  spline S158 degree 3 poles (57.0169, -27.6704) (55.7387, -31.2473) (54.4525, -34.8214) (53.1977, -38.4066) knots 0 0 0 0 1 1 1 1
  spline S159 degree 3 poles (53.1977, -38.4066) (52.7378, -39.7205) (52.2958, -41.0495) (52.3874, -42.4803) knots 0 0 0 0 1 1 1 1
  spline S160 degree 3 poles (52.3874, -42.4803) (52.3929, -42.5673) (52.3208, -42.6844) (52.2494, -42.7473) knots 0 0 0 0 1 1 1 1
  spline S161 degree 3 poles (52.2494, -42.7473) (51.8299, -43.117) (51.4215, -43.505) (50.9682, -43.8296) knots 0 0 0 0 1 1 1 1
  spline S162 degree 3 poles (50.9682, -43.8296) (50.2819, -44.3211) (49.495, -44.5041) (48.6533, -44.4098) knots 0 0 0 0 1 1 1 1
  spline S163 degree 3 poles (48.6533, -44.4098) (48.0159, -44.3384) (47.5969, -43.9415) (47.5472, -43.3015) knots 0 0 0 0 1 1 1 1
  spline S164 degree 3 poles (47.5472, -43.3015) (47.5124, -42.8522) (47.5238, -42.3918) (47.5794, -41.9443) knots 0 0 0 0 1 1 1 1
  spline S165 degree 3 poles (47.5794, -41.9443) (47.7533, -40.5433) (48.1881, -39.2037) (48.6587, -37.8828) knots 0 0 0 0 1 1 1 1
  spline S166 degree 3 poles (48.6587, -37.8828) (50.6099, -32.4064) (52.5864, -26.939) (54.5533, -21.4682) knots 0 0 0 0 1 1 1 1
  spline S167 degree 3 poles (54.5533, -21.4682) (54.7762, -20.8484) (54.9976, -20.2281) (55.2275, -19.5862) knots 0 0 0 0 1 1 1 1
  spline S168 degree 3 poles (55.2275, -19.5862) (55.1098, -19.5785) (55.0374, -19.5698) (54.965, -19.5698) knots 0 0 0 0 1 1 1 1
  spline S169 degree 3 poles (54.965, -19.5698) (53.7273, -19.5691) (52.4896, -19.5659) (51.252, -19.5784) knots 0 0 0 0 1 1 1 1
  spline S170 degree 3 poles (51.252, -19.5784) (51.1737, -19.5792) (51.0605, -19.6886) (51.0256, -19.7731) knots 0 0 0 0 1 1 1 1
  spline S171 degree 3 poles (51.0256, -19.7731) (50.9049, -20.0653) (50.8124, -20.369) (50.7079, -20.6679) knots 0 0 0 0 1 1 1 1
  spline S172 degree 3 poles (50.7079, -20.6679) (50.5007, -21.2605) (50.2927, -21.8528) (50.085, -22.4452) knots 0 0 0 0 1 1 1 1
  line L15 (50.085, -22.4452) -> (50.0849, -22.4452)
  spline S173 degree 3 poles (84.1667, -10.1913) (84.1605, -11.7915) (85.3374, -12.9908) (86.9258, -13.0029) knots 0 0 0 0 1 1 1 1
  spline S174 degree 3 poles (86.9258, -13.0029) (88.5136, -13.0149) (89.7183, -11.8206) (89.7211, -10.2316) knots 0 0 0 0 1 1 1 1
  spline S175 degree 3 poles (89.7211, -10.2316) (89.7239, -8.6369) (88.5314, -7.4321) (86.9503, -7.4324) knots 0 0 0 0 1 1 1 1
  spline S176 degree 3 poles (86.9503, -7.4324) (85.3768, -7.4326) (84.1729, -8.6259) (84.1667, -10.1913) knots 0 0 0 0 1 1 1 1
  spline S177 degree 3 poles (95.1478, -61.341) (95.2089, -61.0965) (95.2508, -60.8445) (95.342, -60.6118) knots 0 0 0 0 1 1 1 1
  spline S178 degree 3 poles (95.342, -60.6118) (95.3717, -60.5363) (95.5302, -60.4704) (95.6303, -60.4696) knots 0 0 0 0 1 1 1 1
  spline S179 degree 3 poles (95.6303, -60.4696) (96.8573, -60.46) (98.0845, -60.4581) (99.3115, -60.4681) knots 0 0 0 0 1 1 1 1
  spline S180 degree 3 poles (99.3115, -60.4681) (99.5329, -60.4699) (99.6414, -60.4125) (99.7194, -60.1902) knots 0 0 0 0 1 1 1 1
  spline S181 degree 3 poles (99.7194, -60.1902) (104.3365, -47.04) (108.9605, -33.8922) (113.5834, -20.7441) knots 0 0 0 0 1 1 1 1
  spline S182 degree 3 poles (113.5834, -20.7441) (113.6177, -20.6465) (113.6473, -20.5473) (113.6878, -20.4221) knots 0 0 0 0 1 1 1 1
  line L16 (113.6878, -20.4221) -> (108.2252, -20.4221)
  spline S183 degree 3 poles (108.2252, -20.4221) (108.2979, -20.1549) (108.3413, -19.9076) (108.4397, -19.6844) knots 0 0 0 0 1 1 1 1
  spline S184 degree 3 poles (108.4397, -19.6844) (108.4711, -19.6131) (108.6477, -19.5743) (108.7581, -19.5739) knots 0 0 0 0 1 1 1 1
  spline S185 degree 3 poles (108.7581, -19.5739) (110.3977, -19.567) (112.0374, -19.5691) (113.677, -19.5691) knots 0 0 0 0 1 1 1 1
  spline S186 degree 3 poles (113.677, -19.5691) (114.9147, -19.5691) (116.1524, -19.5691) (117.39, -19.5691) knots 0 0 0 0 1 1 1 1
  line L17 (117.39, -19.5691) -> (117.794, -19.5691)
  spline S187 degree 3 poles (117.794, -19.5691) (117.3783, -20.8626) (116.9751, -22.1176) (116.5718, -23.3725) knots 0 0 0 0 1 1 1 1
  line L18 (116.5718, -23.3725) -> (116.6331, -23.4021)
  spline S188 degree 3 poles (116.6331, -23.4021) (116.6934, -23.3224) (116.7552, -23.2438) (116.8137, -23.1628) knots 0 0 0 0 1 1 1 1
  spline S189 degree 3 poles (116.8137, -23.1628) (118.1223, -21.3511) (119.7817, -19.9664) (121.9017, -19.2309) knots 0 0 0 0 1 1 1 1
  spline S190 degree 3 poles (121.9017, -19.2309) (125.0975, -18.1221) (129.2488, -19.0142) (131.4403, -22.7614) knots 0 0 0 0 1 1 1 1
  spline S191 degree 3 poles (131.4403, -22.7614) (132.2982, -24.2283) (132.7164, -25.831) (132.9158, -27.5036) knots 0 0 0 0 1 1 1 1
  spline S192 degree 3 poles (132.9158, -27.5036) (133.3231, -30.9198) (132.3382, -34.0053) (130.6312, -36.8985) knots 0 0 0 0 1 1 1 1
  spline S193 degree 3 poles (130.6312, -36.8985) (128.6456, -40.264) (125.9058, -42.8382) (122.343, -44.485) knots 0 0 0 0 1 1 1 1
  spline S194 degree 3 poles (122.343, -44.485) (120.4877, -45.3426) (118.5105, -45.7123) (116.4762, -45.532) knots 0 0 0 0 1 1 1 1
  spline S195 degree 3 poles (116.4762, -45.532) (114.0521, -45.3171) (112.4488, -43.9326) (111.5257, -41.7321) knots 0 0 0 0 1 1 1 1
  spline S196 degree 3 poles (111.5257, -41.7321) (111.3001, -41.1945) (111.1778, -40.6135) (110.9796, -39.9584) knots 0 0 0 0 1 1 1 1
  spline S197 degree 3 poles (110.9796, -39.9584) (108.5658, -46.8189) (106.1753, -53.6131) (103.7692, -60.4516) knots 0 0 0 0 1 1 1 1
  line L19 (103.7692, -60.4516) -> (108.7043, -60.4516)
  spline S198 degree 3 poles (108.7043, -60.4516) (108.6209, -60.7782) (108.5491, -61.0596) (108.4773, -61.341) knots 0 0 0 0 1 1 1 1
  line L20 (108.4773, -61.341) -> (95.1478, -61.341)
  spline S199 degree 3 poles (128.8614, -26.1716) (128.8638, -24.552) (128.6621, -23.2915) (128.1613, -22.0809) knots 0 0 0 0 1 1 1 1
  spline S200 degree 3 poles (128.1613, -22.0809) (127.6838, -20.9266) (126.9085, -20.1109) (125.6676, -19.8061) knots 0 0 0 0 1 1 1 1
  spline S201 degree 3 poles (125.6676, -19.8061) (124.8028, -19.5937) (123.9276, -19.5934) (123.056, -19.7578) knots 0 0 0 0 1 1 1 1
  spline S202 degree 3 poles (123.056, -19.7578) (121.5941, -20.0336) (120.4047, -20.8235) (119.3159, -21.7871) knots 0 0 0 0 1 1 1 1
  spline S203 degree 3 poles (119.3159, -21.7871) (118.185, -22.7878) (117.2705, -23.9794) (116.3717, -25.182) knots 0 0 0 0 1 1 1 1
  spline S204 degree 3 poles (116.3717, -25.182) (116.2291, -25.3728) (116.1079, -25.5914) (116.0281, -25.8153) knots 0 0 0 0 1 1 1 1
  spline S205 degree 3 poles (116.0281, -25.8153) (114.5515, -29.9585) (113.0797, -34.1034) (111.6206, -38.2527) knots 0 0 0 0 1 1 1 1
  spline S206 degree 3 poles (111.6206, -38.2527) (111.5424, -38.4751) (111.5353, -38.7499) (111.5818, -38.983) knots 0 0 0 0 1 1 1 1
  spline S207 degree 3 poles (111.5818, -38.983) (111.687, -39.5095) (111.834, -40.0287) (111.9863, -40.5443) knots 0 0 0 0 1 1 1 1
  spline S208 degree 3 poles (111.9863, -40.5443) (112.3341, -41.7221) (112.9324, -42.7442) (113.845, -43.5861) knots 0 0 0 0 1 1 1 1
  spline S209 degree 3 poles (113.845, -43.5861) (115.4801, -45.0946) (118.0331, -45.0928) (119.806, -44.129) knots 0 0 0 0 1 1 1 1
  spline S210 degree 3 poles (119.806, -44.129) (121.3489, -43.2903) (122.5648, -42.0801) (123.61, -40.6911) knots 0 0 0 0 1 1 1 1
  spline S211 degree 3 poles (123.61, -40.6911) (125.3817, -38.3368) (126.5931, -35.6965) (127.5153, -32.9166) knots 0 0 0 0 1 1 1 1
  spline S212 degree 3 poles (127.5153, -32.9166) (128.276, -30.6235) (128.8153, -28.284) (128.8614, -26.1716) knots 0 0 0 0 1 1 1 1
  spline S213 degree 3 poles (156.0195, -23.5976) (155.9663, -23.8735) (155.9222, -24.1517) (155.8582, -24.4251) knots 0 0 0 0 1 1 1 1
  spline S214 degree 3 poles (155.8582, -24.4251) (155.5238, -25.8533) (154.6088, -26.874) (153.4759, -27.7167) knots 0 0 0 0 1 1 1 1
  spline S215 degree 3 poles (153.4759, -27.7167) (152.0871, -28.7496) (150.5076, -29.403) (148.8648, -29.9105) knots 0 0 0 0 1 1 1 1
  spline S216 degree 3 poles (148.8648, -29.9105) (146.7045, -30.5779) (144.493, -30.9934) (142.2347, -31.0619) knots 0 0 0 0 1 1 1 1
  spline S217 degree 3 poles (142.2347, -31.0619) (141.0145, -31.0989) (139.7894, -30.9729) (138.503, -30.9178) knots 0 0 0 0 1 1 1 1
  spline S218 degree 3 poles (138.503, -30.9178) (138.3184, -31.5134) (138.1099, -32.1735) (137.9094, -32.836) knots 0 0 0 0 1 1 1 1
  spline S219 degree 3 poles (137.0087, -38.7285) (137.0345, -39.7935) (137.1687, -40.8411) (137.642, -41.8068) knots 0 0 0 0 1 1 1 1
  spline S220 degree 3 poles (137.642, -41.8068) (138.4938, -43.5447) (139.955, -44.4468) (141.8277, -44.718) knots 0 0 0 0 1 1 1 1
  spline S221 degree 3 poles (141.8277, -44.718) (144.246, -45.0682) (146.3193, -44.2615) (148.1741, -42.7628) knots 0 0 0 0 1 1 1 1
  spline S222 degree 3 poles (148.1741, -42.7628) (149.3448, -41.8167) (150.286, -40.6676) (151.1384, -39.4379) knots 0 0 0 0 1 1 1 1
  spline S223 degree 3 poles (151.1384, -39.4379) (151.3182, -39.1785) (151.52, -38.9343) (151.7296, -38.6596) knots 0 0 0 0 1 1 1 1
  spline S224 degree 3 poles (151.7296, -38.6596) (151.9691, -38.7968) (152.1937, -38.9254) (152.41, -39.0493) knots 0 0 0 0 1 1 1 1
  spline S225 degree 3 poles (152.41, -39.0493) (151.1962, -41.1095) (149.6959, -42.8569) (147.6206, -44.0951) knots 0 0 0 0 1 1 1 1
  spline S226 degree 3 poles (147.6206, -44.0951) (145.4638, -45.3818) (143.1519, -45.7339) (140.7013, -45.5057) knots 0 0 0 0 1 1 1 1
  spline S227 degree 3 poles (140.7013, -45.5057) (138.6131, -45.3113) (136.8021, -44.5156) (135.3221, -43.0231) knots 0 0 0 0 1 1 1 1
  spline S228 degree 3 poles (135.3221, -43.0231) (133.9884, -41.6782) (133.2638, -40.0236) (132.9818, -38.1701) knots 0 0 0 0 1 1 1 1
  spline S229 degree 3 poles (132.9818, -38.1701) (132.6126, -35.7441) (133.1018, -33.4352) (134.0532, -31.2182) knots 0 0 0 0 1 1 1 1
  spline S230 degree 3 poles (134.0532, -31.2182) (136.0205, -26.6341) (139.1004, -23.0008) (143.4312, -20.4739) knots 0 0 0 0 1 1 1 1
  spline S231 degree 3 poles (143.4312, -20.4739) (145.5366, -19.2454) (147.8053, -18.6354) (150.2562, -18.8437) knots 0 0 0 0 1 1 1 1
  spline S232 degree 3 poles (150.2562, -18.8437) (151.8701, -18.9809) (153.4053, -19.3719) (154.6851, -20.4397) knots 0 0 0 0 1 1 1 1
  spline S233 degree 3 poles (154.6851, -20.4397) (155.4188, -21.052) (155.8891, -21.8192) (155.9685, -22.7942) knots 0 0 0 0 1 1 1 1
  spline S234 degree 3 poles (155.9685, -22.7942) (155.9715, -22.8305) (156.0019, -22.8646) (156.0195, -22.8998) knots 0 0 0 0 1 1 1 1
  line L21 (156.0195, -22.8998) -> (156.0195, -23.5976)
  spline S235 degree 3 poles (138.7712, -30.0038) (139.2833, -30.0649) (139.7002, -30.1254) (140.1191, -30.1628) knots 0 0 0 0 1 1 1 1
  spline S236 degree 3 poles (140.1191, -30.1628) (142.2832, -30.356) (144.4026, -30.1915) (146.4395, -29.3662) knots 0 0 0 0 1 1 1 1
  spline S237 degree 3 poles (146.4395, -29.3662) (148.2949, -28.6145) (149.935, -27.569) (151.122, -25.9174) knots 0 0 0 0 1 1 1 1
  spline S238 degree 3 poles (151.122, -25.9174) (151.9809, -24.7224) (152.4727, -23.4101) (152.2726, -21.9102) knots 0 0 0 0 1 1 1 1
  spline S239 degree 3 poles (152.2726, -21.9102) (152.1161, -20.7367) (151.3327, -19.8797) (150.1687, -19.7408) knots 0 0 0 0 1 1 1 1
  spline S240 degree 3 poles (150.1687, -19.7408) (149.4761, -19.6581) (148.7512, -19.6761) (148.0608, -19.7806) knots 0 0 0 0 1 1 1 1
  spline S241 degree 3 poles (148.0608, -19.7806) (146.7386, -19.9808) (145.6448, -20.6992) (144.619, -21.5155) knots 0 0 0 0 1 1 1 1
  spline S242 degree 3 poles (144.619, -21.5155) (142.6739, -23.0631) (141.2378, -25.0227) (140.0927, -27.2034) knots 0 0 0 0 1 1 1 1
  spline S243 degree 3 poles (140.0927, -27.2034) (139.6235, -28.0968) (139.2283, -29.0291) (138.7712, -30.0038) knots 0 0 0 0 1 1 1 1
  spline S244 degree 3 poles (50.0849, -22.4452) (50.2926, -21.8528) (50.5007, -21.2605) (50.7079, -20.6679) knots 0 0 0 0 1 1 1 1
  spline S245 degree 3 poles (50.7079, -20.6679) (50.8123, -20.369) (50.9049, -20.0653) (51.0255, -19.7731) knots 0 0 0 0 1 1 1 1
  spline S246 degree 3 poles (51.0255, -19.7731) (51.0604, -19.6886) (51.1737, -19.5792) (51.252, -19.5784) knots 0 0 0 0 1 1 1 1
  spline S247 degree 3 poles (51.252, -19.5784) (52.4895, -19.5659) (53.7273, -19.5691) (54.965, -19.5698) knots 0 0 0 0 1 1 1 1
  spline S248 degree 3 poles (54.965, -19.5698) (55.0374, -19.5698) (55.1098, -19.5785) (55.2275, -19.5862) knots 0 0 0 0 1 1 1 1
  spline S249 degree 3 poles (55.2275, -19.5862) (54.9976, -20.2281) (54.7762, -20.8484) (54.5533, -21.4682) knots 0 0 0 0 1 1 1 1
  spline S250 degree 3 poles (54.5533, -21.4682) (52.5863, -26.939) (50.6099, -32.4064) (48.6587, -37.8828) knots 0 0 0 0 1 1 1 1
  spline S251 degree 3 poles (48.6587, -37.8828) (48.188, -39.2037) (47.7533, -40.5433) (47.5793, -41.9443) knots 0 0 0 0 1 1 1 1
  spline S252 degree 3 poles (47.5793, -41.9443) (47.5238, -42.3918) (47.5124, -42.8522) (47.5472, -43.3015) knots 0 0 0 0 1 1 1 1
  spline S253 degree 3 poles (47.5472, -43.3015) (47.5969, -43.9415) (48.0158, -44.3384) (48.6532, -44.4098) knots 0 0 0 0 1 1 1 1
  spline S254 degree 3 poles (48.6532, -44.4098) (49.495, -44.5041) (50.2819, -44.3211) (50.9682, -43.8296) knots 0 0 0 0 1 1 1 1
  spline S255 degree 3 poles (50.9682, -43.8296) (51.4214, -43.505) (51.8299, -43.117) (52.2494, -42.7473) knots 0 0 0 0 1 1 1 1
  spline S256 degree 3 poles (52.2494, -42.7473) (52.3208, -42.6843) (52.3929, -42.5673) (52.3873, -42.4803) knots 0 0 0 0 1 1 1 1
  spline S257 degree 3 poles (52.3873, -42.4803) (52.2958, -41.0495) (52.7378, -39.7205) (53.1976, -38.4066) knots 0 0 0 0 1 1 1 1
  spline S258 degree 3 poles (53.1976, -38.4066) (54.4524, -34.8214) (55.7386, -31.2473) (57.0169, -27.6704) knots 0 0 0 0 1 1 1 1
  spline S259 degree 3 poles (57.0169, -27.6704) (60.1698, -18.8474) (63.3253, -10.0253) (66.4793, -1.2026) knots 0 0 0 0 1 1 1 1
  spline S260 degree 3 poles (66.4793, -1.2026) (66.5105, -1.1153) (66.5356, -1.0258) (66.5753, -0.8998) knots 0 0 0 0 1 1 1 1
  line L22 (66.5753, -0.8998) -> (61.3495, -0.8998)
  spline S261 degree 3 poles (61.3495, -0.8998) (61.434, -0.5992) (61.5071, -0.3392) (61.5817, -0.0737) knots 0 0 0 0 1 1 1 1
  line L23 (61.5817, -0.0737) -> (70.961, -0.0737)
  spline S262 degree 3 poles (70.961, -0.0737) (70.9285, -0.1807) (70.9037, -0.2765) (70.8707, -0.3694) knots 0 0 0 0 1 1 1 1
  spline S263 degree 3 poles (70.8707, -0.3694) (66.7267, -12.0314) (62.5801, -23.6925) (58.4397, -35.3559) knots 0 0 0 0 1 1 1 1
  spline S264 degree 3 poles (58.4397, -35.3559) (57.7268, -37.364) (57.0232, -39.3758) (56.3538, -41.3985) knots 0 0 0 0 1 1 1 1
  spline S265 degree 3 poles (56.3538, -41.3985) (56.1806, -41.9219) (56.0896, -42.4913) (56.0712, -43.0432) knots 0 0 0 0 1 1 1 1
  spline S266 degree 3 poles (56.0712, -43.0432) (56.0306, -44.2662) (56.8851, -44.9938) (58.0846, -44.749) knots 0 0 0 0 1 1 1 1
  spline S267 degree 3 poles (58.0846, -44.749) (58.5682, -44.6503) (59.0639, -44.4504) (59.4731, -44.176) knots 0 0 0 0 1 1 1 1
  spline S268 degree 3 poles (59.4731, -44.176) (61.1119, -43.0774) (62.2985, -41.5649) (63.1257, -39.7979) knots 0 0 0 0 1 1 1 1
  spline S269 degree 3 poles (63.1257, -39.7979) (63.6148, -38.7533) (63.951, -37.6361) (64.3408, -36.5461) knots 0 0 0 0 1 1 1 1
  spline S270 degree 3 poles (64.3408, -36.5461) (68.5443, -24.7933) (72.7448, -13.0394) (76.9459, -1.2857) knots 0 0 0 0 1 1 1 1